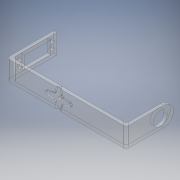
# Autodesk Inventor part: outerGantry
Saved by Autodesk Inventor 2018 (Build 220112000, 112)
## iProperties
Created: 2017-07-30
Part Number: outerGantry
Material: PET Plastic
Document SubType Name: Modeling
Designer: kurtis
Density: 1.541 g/cm^3
Appearance: Polycarbonate - Clear
Author: kurtis
Autodesk Inventor part; units mm, degrees
ref_plane "YZ Plane" through (0, 0, 0) normal (1, 0, 0) x (0, 1, 0)
ref_plane "XZ Plane" through (0, 0, 0) normal (0, 1, 0) x (-1, 0, 0)
ref_plane "XY Plane" through (0, 0, 0) normal (0, 0, 1) x (1, 0, 0)
sketch "Sketch1" plane through (0, 0, 0) normal (0, 0, 1) x (1, 0, 0)
  line L0 (0, 0) -> (175, 0)
  line L1 (0, 0) -> (0, 68)
  line L2 (0, 68) -> (-5, 68)
  line L3 (-5, 68) -> (-5, -5)
  line L4 (-5, -5) -> (180, -5)
  line L5 (180, -5) -> (180, 68)
  line L6 (180, 68) -> (175, 68)
  line L7 (175, 68) -> (175, 0)
  dimension "d0" = 175
  dimension "d1" = 68
  dimension "d2" = 5
  dimension "d3" = 73
  dimension "d4" = 185
  dimension "d5" = 73
  dimension "d6" = 5
  constraints: 16 end point, 3 vertical, 2 horizontal, 2 perpendicular
  measures "d0" distance of L0.start L0.end
  measures "d1" distance of L0.start L1.end
  measures "d2" distance of L1.end L2.end
  measures "d3" distance of L2.end L3.end
  measures "d4" distance of L3.end L4.end
  measures "d5" distance of L4.end L5.end
  measures "d6" distance of L5.end L6.end
extrude "Outline" add sketch "Sketch1" along normal blind 30
sketch "Sketch2" plane through (-5, -5, 0) normal (-1, 0, 0) x (0, 0, 1)
  line L0 (0, 73) -> (30, 73) construction
  line L1 (15, 73) -> (15, 43) construction
  line L2 (5, 22.5) -> (25, 22.5)
  line L3 (25, 22.5) -> (25, 63.5)
  line L4 (25, 63.5) -> (5, 63.5)
  line L5 (5, 63.5) -> (5, 22.5)
  line L6 (5, 22.5) -> (25, 63.5) construction
  line L7 (25, 22.5) -> (5, 63.5) construction
  line L8 (5, 63.5) -> (5, 67.5) construction
  line L9 (5, 67.5) -> (10, 67.5) construction
  line L10 (25, 63.5) -> (25, 67.5) construction
  line L11 (25, 67.5) -> (20, 67.5) construction
  line L12 (5, 22.5) -> (5, 18.5) construction
  line L13 (5, 18.5) -> (10, 18.5) construction
  line L14 (25, 22.5) -> (25, 18.5) construction
  line L15 (25, 18.5) -> (20, 18.5) construction
  circle A0 centre (10, 67.5) radius 2
  circle A1 centre (20, 67.5) radius 2
  circle A2 centre (10, 18.5) radius 2
  circle A3 centre (20, 18.5) radius 2
  point P0 (0, 5)
  dimension "d9" = 30
  dimension "d10" = 20
  dimension "d11" = 41
  dimension "d12" = 4
  dimension "d13" = 5
  dimension "d14" = 4
  dimension "d15" = 5
  dimension "d16" = 4
  dimension "d17" = 5
  dimension "d18" = 4
  dimension "d19" = 5
  dimension "d20" = 4
  dimension "d21" = 4
  dimension "d22" = 4
  dimension "d23" = 4
  constraints: 30 end point, 5 perpendicular, 5 vertical, 4 centre point, 4 coincident, 3 midpoint, 2 parallel, 1 horizontal
  measures "d9" distance of L1.start L1.end
  measures "d10" distance of L4.end L3.end
  measures "d11" distance of L3.end L2.end
  measures "d12" distance of L4.end L8.end
  measures "d13" distance of L8.end L9.end
  measures "d14" distance of L3.end L10.end
  measures "d15" distance of L10.end L11.end
  measures "d16" distance of L2.start L12.end
  measures "d17" distance of L12.end L13.end
  measures "d18" distance of L2.end L14.end
  measures "d19" distance of L14.end L15.end
  measures "d20" diameter of A0
  measures "d21" diameter of A1
  measures "d22" diameter of A2
  measures "d23" diameter of A3
extrude "Servo Mount" cut sketch "Sketch2" against normal blind 10
sketch "Sketch3" plane through (175, 0, 0) normal (-1, 0, 0) x (0, 0, 1)
  line L0 (5, 58.5) -> (25, 58.5) construction
  line L1 (15, 58.5) -> (15, 47.5) construction
  circle A0 centre (15, 47.5) radius 10.75
  point P0 (0, 0)
  dimension "d26" = 11
  dimension "d27" = 21.5
  constraints: 2 end point, 1 centre point, 1 coincident, 1 midpoint, 1 vertical
  measures "d26" distance of L1.start L1.end
  measures "d27" diameter of A0
extrude "Idler Mount" cut sketch "Sketch3" against normal blind 14.5
sketch "Sketch4" plane through (-5, -5, 0) normal (0, -1, 0) x (1, 0, 0)
  line L0 (0, 25) -> (0, 5) construction
  line L1 (99.5, 14.2941) -> (99.5, 15.7059)
  line L2 (60.5, 15.7059) -> (60.5, 14.2941)
  line L3 (79.2941, 34.5) -> (80.7059, 34.5)
  line L4 (80.7059, -4.5) -> (79.2941, -4.5)
  line L5 (84.5, 22.5) -> (84.5, 21.5)
  line L6 (84.5, 8.5) -> (84.5, 7.5)
  line L7 (75.5, 7.5) -> (75.5, 8.5)
  line L8 (75.5, 21.5) -> (75.5, 22.5)
  line L9 (72.5, 10.5) -> (73.5, 10.5)
  line L10 (86.5, 10.5) -> (87.5, 10.5)
  line L11 (87.5, 19.5) -> (86.5, 19.5)
  line L12 (73.5, 19.5) -> (72.5, 19.5)
  arc A0 (73.5, 19.5) -> (75.5, 21.5) centre (73.5, 21.5) ccw
  arc A1 (84.5, 21.5) -> (86.5, 19.5) centre (86.5, 21.5) ccw
  arc A2 (86.5, 10.5) -> (84.5, 8.5) centre (86.5, 8.5) ccw
  arc A3 (75.5, 8.5) -> (73.5, 10.5) centre (73.5, 8.5) ccw
  line L13 (84.5, 22.5) -> (82.6755, 32.8473)
  line L14 (75.5, 22.5) -> (77.3245, 32.8473)
  line L15 (87.5, 10.5) -> (97.8473, 12.3245)
  line L16 (87.5, 19.5) -> (97.8473, 17.6755)
  line L17 (72.5, 19.5) -> (62.1527, 17.6755)
  line L18 (72.5, 10.5) -> (62.1527, 12.3245)
  line L19 (75.5, 7.5) -> (77.3245, -2.8473)
  line L20 (84.5, 7.5) -> (82.6755, -2.8473)
  arc A4 (62.1527, 17.6755) -> (60.5, 15.7059) centre (62.5, 15.7059) ccw
  arc A5 (60.5, 14.2941) -> (62.1527, 12.3245) centre (62.5, 14.2941) ccw
  arc A6 (79.2941, 34.5) -> (77.3245, 32.8473) centre (79.2941, 32.5) ccw
  arc A7 (82.6755, 32.8473) -> (80.7059, 34.5) centre (80.7059, 32.5) ccw
  arc A8 (99.5, 15.7059) -> (97.8473, 17.6755) centre (97.5, 15.7059) ccw
  arc A9 (97.8473, 12.3245) -> (99.5, 14.2941) centre (97.5, 14.2941) ccw
  arc A10 (77.3245, -2.8473) -> (79.2941, -4.5) centre (79.2941, -2.5) ccw
  arc A11 (80.7059, -4.5) -> (82.6755, -2.8473) centre (80.7059, -2.5) ccw
  line L21 (80, 15) -> (66, 15) construction
  line L22 (80, 15) -> (80, 29) construction
  line L23 (80, 15) -> (94, 15) construction
  line L24 (80, 15) -> (80, 1) construction
  circle A12 centre (80, 29) radius 0.75
  circle A13 centre (66, 15) radius 0.75
  circle A14 centre (94, 15) radius 0.75
  circle A15 centre (80, 1) radius 0.75
  circle A16 centre (80, 15) radius 2.5
  point P0 (5, 0)
  dimension "d35" = 2
  dimension "d37" = 10
  dimension "d39" = 10
  dimension "d41" = 10
  dimension "d43" = 10
  dimension "d45" = 10
  dimension "d47" = 10
  dimension "d49" = 10
  dimension "d51" = 10
  dimension "d52" = 2
  dimension "d53" = 2
  dimension "d54" = 80
  dimension "d55" = 6.5
  dimension "d56" = 6.5
  dimension "d57" = 14
  dimension "d58" = 14
  dimension "d59" = 14
  dimension "d60" = 14
  dimension "d61" = 1.5
  dimension "d62" = 1.5
  dimension "d63" = 1.5
  dimension "d64" = 1.5
  dimension "d70" = 5
  constraints: 48 end point, 28 tangent, 24 point on circle, 17 centre point, 10 parallel, 9 equal radius, 6 coincident, 5 horizontal, 4 perpendicular, 2 vertical
  measures "d35" radius of A0
  measures "d37" angle of L5 L13
  measures "d39" angle of L8 L14
  measures "d41" angle of L10 L15
  measures "d43" angle of L11 L16
  measures "d45" angle of L12 L17
  measures "d47" angle of L9 L18
  measures "d49" angle of L7 L19
  measures "d51" angle of L6 L20
  measures "d52" radius of A4
  measures "d53" radius of A6
  measures "d54" distance from line of point (80, 15) L0
  measures "d55" horizontal distance of point (80, 15) A0.centre
  measures "d56" horizontal distance of point (80, 15) A0.centre
  measures "d57" distance of L21.start L21.end
  measures "d58" distance of L21.start L22.end
  measures "d59" distance of L21.start L23.end
  measures "d60" distance of L21.start L24.end
  measures "d61" diameter of A12
  measures "d62" diameter of A13
  measures "d63" diameter of A14
  measures "d64" diameter of A15
  measures "d70" diameter of A16
extrude "Bottom Servo indent" cut sketch "Sketch4" against normal blind 2 contours A9 L15 L10 A2 L6 L20 A11 L4 A10 L19 L7 A3 L9 L18 A5 L2 A4 L17 L12 A0 L8 L14 A6 L3 A7 L13 L5 A1 L11 L16 A8 L1 | A16
extrude "Bottom Servo Mounting Holse" cut sketch "Sketch4" against normal blind 22 contours A12 | A13 | A14 | A15 | A16
fillet "Strengthening Fillet" radius 4 4 edges at (0, 0, 15) (175, 0, 15) (-5, -5, 15) (180, -5, 15)
fillet "Rounded Idler Post" radius 15 2 edges at (177.5, 68, 0) (177.5, 68, 30)
equation "\"d3\" = d1 + d2"
equation "\"d4\" = d0 + 2 * d2"
equation "\"d5\" = d3"
equation "\"d6\" = d2"
equation "\"d14\" = d12"
equation "\"d15\" = d13"
equation "\"d16\" = d12"
equation "\"d17\" = d13"
equation "\"d18\" = d12"
equation "\"d19\" = d13"
equation "\"d39\" = d37"
equation "\"d41\" = d37"
equation "\"d43\" = d37"
equation "\"d45\" = d37"
equation "\"d47\" = d37"
equation "\"d49\" = d37"
equation "\"d51\" = d37"
equation "\"d58\" = d57"
equation "\"d59\" = d57"
equation "\"d60\" = d57"
equation "\"d62\" = d61"
equation "\"d63\" = d61"
equation "\"d64\" = d61"
body "Solid1"
